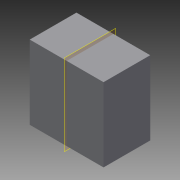
# Autodesk Inventor part: camera
Saved by Autodesk Inventor 2014 (Build 180170000, 170)
## iProperties
Created: 2013-09-08
Part Number: camera
Material: Generisch
Document SubType Name: Modeling
Designer: Felix
Density: 1 g/cm^3
Appearance: Vorgabe
Mass: 0.31205 g
Surface Area: 2.8282 cm^2
Volume: 0.31205 cm^3
Author: Felix
Autodesk Inventor part; units mm, degrees
ref_plane "YZ Plane" through (0, 0, 0) normal (1, 0, 0) x (0, 1, 0)
ref_plane "XZ Plane" through (0, 0, 0) normal (0, 1, 0) x (-1, 0, 0)
ref_plane "XY Plane" through (0, 0, 0) normal (0, 0, 1) x (1, 0, 0)
sketch "Skizze1" plane through (0, 0, 0) normal (0, 1, 0) x (-1, 0, 0)
  line L0 (0, 0) -> (7.9, 0)
  line L1 (7.9, 0) -> (7.9, 7.9)
  line L2 (7.9, 7.9) -> (0, 7.9)
  line L3 (0, 7.9) -> (0, 0)
  dimension "d0" = 7.9
  dimension "d1" = 7.9
  constraints: 8 end point, 2 parallel, 1 horizontal, 1 perpendicular
  measures "d0" distance of L2.end L1.end
  measures "d1" distance of L1.end L0.end
extrude "Extrusion1" add sketch "Skizze1" along normal blind 5
ref_plane "Arbeitsebene1" through (-3.95, 5, 7.9) normal (1, 0, 0) x (0, 0, -1)
